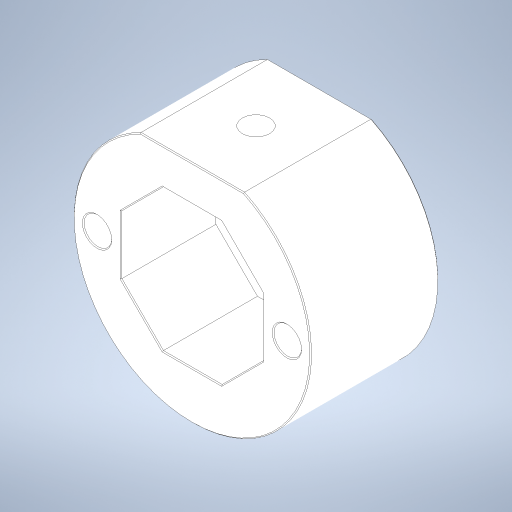
# Autodesk Inventor part: spool_center
Saved by Autodesk Inventor 2023 (Build 270158000, 158)
## iProperties
Created: 2023-11-23
Part Number: spool_center
Material: Generic
Document SubType Name: Modeling
Designer: aaron
Density: 1 g/cm^3
Appearance: Default
Author: aaron
Autodesk Inventor part; units mm, degrees
ref_plane "YZ Plane" through (0, 0, 0) normal (1, 0, 0) x (0, 1, 0)
ref_plane "XZ Plane" through (0, 0, 0) normal (0, 1, 0) x (-1, 0, 0)
ref_plane "XY Plane" through (0, 0, 0) normal (0, 0, 1) x (1, 0, 0)
sketch "Sketch2" plane through (0, 0, 0) normal (0, 0, 1) x (1, 0, 0)
  circle A0 centre (0, 0) radius 25
  line L0 (-17.0079, 22.5) -> (27.1684, 22.5)
  point P0 (10.8972, 22.5)
  point P1 (-10.8972, 22.5)
  dimension "d4" = 50
  dimension "d5" = 22.5
  constraints: 2 end point, 1 centre point, 1 coincident, 1 horizontal
  measures "d4" diameter of A0
  measures "d5" distance from line of L0 A0.centre
extrude "Extrusion2" add sketch "Sketch2" along normal blind 27 contours A0 L0 picked at (1.1654, 4.7055)
sketch "Sketch3" plane through (-10.8972, 22.5, 0) normal (0, 1, 0) x (1, 0, 0)
  circle A0 centre (10.8972, -13.5) radius 2.875
  line L0 (0, 0) -> (0, -27) projected
  line L1 (21.7945, 0) -> (21.7945, -27) projected
  line L2 (21.7945, 0) -> (0, 0) projected
  point P0 (10.8972, 0)
  dimension "d8" = 5.75
  dimension "d9" = 10.8972
  dimension "d10" = 21.7945
  dimension "d11" = 27
  dimension "d12" = 13.5
  constraints: 1 centre point
  measures "d8" diameter of A0
  measures "d9" distance from line of L0 A0.centre
  measures "d10" distance between parallel lines of L0 L1
  measures "d11" distance of L1.start L1.end
  measures "d12" distance from line of L2 A0.centre
extrude "Extrusion3" cut sketch "Sketch3" against normal blind 15
sketch "Sketch4" plane through (0, 0, 27) normal (0, 0, 1) x (1, 0, 0)
  line L0 (6.2132, -15) -> (15, -6.2132)
  line L1 (-6.2132, -15) -> (6.2132, -15)
  line L2 (-15, -6.2132) -> (-6.2132, -15)
  line L3 (-15, 6.2132) -> (-15, -6.2132)
  line L4 (-6.2132, 15) -> (-15, 6.2132)
  line L5 (6.2132, 15) -> (-6.2132, 15)
  line L6 (15, 6.2132) -> (6.2132, 15)
  line L7 (15, -6.2132) -> (15, 6.2132)
  line L8 (-6.1884, 14.94) -> (6.1884, 14.94)
  line L9 (6.1884, 14.94) -> (14.94, 6.1884)
  line L10 (14.94, 6.1884) -> (14.94, -6.1884)
  line L11 (14.94, -6.1884) -> (6.1884, -14.94)
  line L12 (6.1884, -14.94) -> (-6.1884, -14.94)
  line L13 (-6.1884, -14.94) -> (-14.94, -6.1884)
  line L14 (-14.94, -6.1884) -> (-14.94, 6.1884)
  line L15 (-14.94, 6.1884) -> (-6.1884, 14.94)
  point P0 (0, 0)
  point P1 (0, 0)
  dimension "d47" = 29.88
  dimension "d48" = 14.94
  dimension "d49" = 14.94
  dimension "d50" = 29.88
  constraints: 32 end point, 3 parallel, 7 other
  measures "d47" distance between parallel lines of L12 L8
  measures "d48" distance from line of L8 point (0, 0)
  measures "d49" distance from line of point (0, 0) L14
  measures "d50" distance between parallel lines of L11 L15
extrude "Extrusion4" cut sketch "Sketch4" against normal blind 20 contours L8 L9 L10 L11 L12 L13 L14 L15
sketch "Sketch6" plane through (0, 0, 27) normal (0, 0, 1) x (1, 0, 0)
  line L0 (-15.1, 6.2546) -> (-6.2546, 15.1) projected
  line L1 (-15.1, -6.2546) -> (-15.1, 6.2546) projected
  line L2 (-6.2546, -15.1) -> (-15.1, -6.2546) projected
  line L3 (6.2546, -15.1) -> (-6.2546, -15.1) projected
  line L4 (15.1, -6.2546) -> (6.2546, -15.1) projected
  line L5 (15.1, 6.2546) -> (15.1, -6.2546) projected
  line L6 (6.2546, 15.1) -> (15.1, 6.2546) projected
  line L7 (-6.2546, 15.1) -> (6.2546, 15.1) projected
  line L8 (0, 0) -> (33.369, 0)
  circle A0 centre (0, 0) radius 20
  circle A1 centre (20, 0) radius 2.9
  circle A2 centre (-20, 0) radius 2.9
  dimension "d20" = 40
  dimension "d21" = 5.8
  dimension "d24" = 360
  constraints: 2 centre point, 2 end point, 1 coincident, 1 horizontal, 1 horizontal alignment, 1 point on line, 7 other
  measures "d21" diameter of A1
extrude "Extrusion6" cut sketch "Sketch6" against normal blind 7 contours A1 A0 L8 | L8 A0 A1 | A0 A1 L8 | L8 A1 A0 | A2 A0 | A0 A2
sketch "Sketch7" plane through (0, 0, 0) normal (0, 0, -1) x (-1, 0, 0)
  line L0 (0, 0) -> (41.4197, 0)
  circle A0 centre (20, 0) radius 2.9 projected
  circle A1 centre (20, 0) radius 2.9
  circle A2 centre (14.1421, 14.1421) radius 2.9
  circle A3 centre (0, 20) radius 2.9
  circle A4 centre (-14.1421, 14.1421) radius 2.9
  circle A5 centre (-20, 0) radius 2.9
  circle A6 centre (-14.1421, -14.1421) radius 2.9
  circle A7 centre (0, -20) radius 2.9
  circle A8 centre (14.1421, -14.1421) radius 2.9
  dimension "d30" = 360
  constraints: 8 centre point, 2 end point, 1 coincident, 1 concentric, 1 horizontal, 17 other
extrude "Extrusion7" cut sketch "Sketch7" against normal blind 10 contours A0 L0 | L0 A0 | A2 | A4 | A5 | A6 | A7 | A8
sketch "Sketch8" plane through (0, 0, 7) normal (0, 0, 1) x (1, 0, 0)
  line L0 (-15.1, 6.2546) -> (-6.2546, 15.1) projected
  line L1 (-15.1, -6.2546) -> (-15.1, 6.2546) projected
  line L2 (-6.2546, -15.1) -> (-15.1, -6.2546) projected
  line L3 (6.2546, -15.1) -> (-6.2546, -15.1) projected
  line L4 (15.1, -6.2546) -> (6.2546, -15.1) projected
  line L5 (15.1, 6.2546) -> (15.1, -6.2546) projected
  line L6 (6.2546, 15.1) -> (15.1, 6.2546) projected
  line L7 (-6.2546, 15.1) -> (6.2546, 15.1) projected
  line L8 (3.7693, 9.1) -> (9.1, 3.7693)
  line L9 (9.1, 3.7693) -> (9.1, -3.7693)
  line L10 (9.1, -3.7693) -> (3.7693, -9.1)
  line L11 (3.7693, -9.1) -> (-3.7693, -9.1)
  line L12 (-3.7693, -9.1) -> (-9.1, -3.7693)
  line L13 (-9.1, -3.7693) -> (-9.1, 3.7693)
  line L14 (-9.1, 3.7693) -> (-3.7693, 9.1)
  line L15 (-3.7693, 9.1) -> (3.7693, 9.1)
  point P0 (0, 0)
  dimension "d34" = 6
  constraints: 16 end point, 7 other
  measures "d34" distance between parallel lines of L7 L15
extrude "Extrusion8" cut sketch "Sketch8" against normal through all contours L8 L9 L10 L11 L12 L13 L14 L15
chamfer "Chamfer1" distance 0.2 angle 45 8 edges at (9.1, 0, 0) (6.4347, 6.4347, 0) (0, 9.1, 0) (-6.4347, 6.4347, 0) (-9.1, 0, 0) (-6.4347, -6.4347, 0) (0, -9.1, 0) (6.4347, -6.4347, 0)
chamfer "Chamfer2" distance 0.2 angle 45 9 edges at (17.0421, 14.1421, 0) (-11.2421, 14.1421, 0) (-17.1, 0, 0) (-11.2421, -14.1421, 0) (2.9, -20, 0) (17.0421, -14.1421, 0) (22.9, 0, 0) (-22.9, 0, 27) (17.1, 0, 27)
chamfer "Chamfer3" distance 0.2 angle 45 4 edges at (0, -25, 0) (0, 22.5, 0) (0, -25, 27) (0, 22.5, 27)
chamfer "Chamfer4" distance 0.2 angle 45 8 edges at (0, 14.94, 27) (10.5642, 10.5642, 27) (14.94, 0, 27) (10.5642, -10.5642, 27) (0, -14.94, 27) (-10.5642, -10.5642, 27) (-14.94, 0, 27) (-10.5642, 10.5642, 27)
equation "\"d9\" = 0.5 * d10"
equation "\"d12\" = 0.5 * d11"
equation "\"d48\" = 0.5 * d47"
equation "\"d49\" = 0.5 * d47"
equation "\"d50\" = d47"
body "Solid2"
